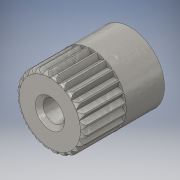
# Autodesk Inventor part: MicroServo Horn
Saved by Autodesk Inventor 2016 (Build 200138000, 138)
## iProperties
Created: 2016-02-12
Part Number: MicroServo Horn
Material: Generic
Document SubType Name: Modeling
Designer: RoksBot
Density: 1 g/cm^3
Appearance: Galvanized
Author: RoksBot
Autodesk Inventor part; units mm, degrees
ref_plane "YZ Plane" through (0, 0, 0) normal (1, 0, 0) x (0, 1, 0)
ref_plane "XZ Plane" through (0, 0, 0) normal (0, 1, 0) x (-1, 0, 0)
ref_plane "XY Plane" through (0, 0, 0) normal (0, 0, 1) x (1, 0, 0)
sketch "Sketch1" plane through (0, 0, 0) normal (0, 0, 1) x (1, 0, 0)
  circle A0 centre (0, 0) radius 2.2733
  dimension "d0" = 4.5466
  constraints: 1 centre point, 1 coincident
  measures "d0" diameter of A0
extrude "Extrusion1" add sketch "Sketch1" along normal blind 5.3086
sketch "Sketch2" plane through (0, 0, 5.3086) normal (0, 0, 1) x (1, 0, 0)
  circle A0 centre (0, 0) radius 0.7112
  dimension "d3" = 1.4224
  constraints: 1 centre point, 1 coincident
  measures "d3" diameter of A0
extrude "Extrusion2" cut sketch "Sketch2" against normal blind 2.7686
chamfer "Chamfer1" distance 0.254 angle 45 1 edges at (-0.7112, 0, 5.3086)
fillet "Fillet1" radius 0.254 1 edges at (-2.2733, 0, 5.3086)
sketch "Sketch3" plane through (0, 0, 5.3086) normal (0, 0, 1) x (1, 0, 0)
  circle A0 centre (0, 0) radius 2.2733 projected
  circle A1 centre (0, 0) radius 2.2733 projected
  line L0 (-0.254, 2.2591) -> (0, 2.0051)
  line L1 (0, 2.0051) -> (0.254, 2.2591)
  dimension "d10" = 0.508
  dimension "d11" = 0.254
  constraints: 4 end point, 4 point on circle, 1 perpendicular, 1 vertical alignment
  measures "d10" distance of L1.end L0.start
  measures "d11" horizontal distance of L1.end L0.end
extrude "Extrusion3" cut sketch "Sketch3" against normal blind 2.7686 contours L1 L0 A0 picked at (0.1129, 2.1786)
pattern_circular "Circular Pattern1" count 24 over 360 about axis through (0, 0, 0) along (0, 0, 1) of "Extrusion3"
body "Solid1"
